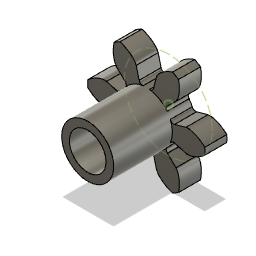
shelf (joined) v52 (Autodesk Fusion 360 archive; units mm, degrees)
design "gear(small)left"
description: small size, for left
description: Spur Gear; Module: 2.0; Num Teeth: 6; Pressure Angle: 20.0; Backlash: 0.00 mm
Autodesk Fusion 360 part; units mm, degrees
(part 1 of 4)
sketch "草图1" plane through (0, 0, 0) normal (0, 0, 1) x (1, 0, 0) in component "Spur Gear (6 teeth)"
  circle A0 centre (0, 0) radius 3.5492
  circle A1 centre (0, 0) radius 2.5
extrude "拉伸1" add sketch "草图1" along normal blind 11 in component "Spur Gear (6 teeth)"
sketch "草图2" plane through (0, 0, 0) normal (0, 0, 1) x (1, 0, 0) in component "Spur Gear (6 teeth)"
  spline S0 degree 5 poles (5.4237, -1.5403) (5.4306, -1.5422) (5.4444, -1.5458) (5.4654, -1.5503) (5.4937, -1.5547) (5.5295, -1.5577) (5.5656, -1.5592) (5.602, -1.5596) (5.6385, -1.5595) (5.6751, -1.559) (5.7117, -1.558) (5.7485, -1.5565) (5.7854, -1.5541) (5.8224, -1.5509) (5.8596, -1.5469) (5.8968, -1.542) (5.9342, -1.5365) (5.9716, -1.5304) (6.009, -1.5238) (6.0465, -1.5167) (6.084, -1.509) (6.1216, -1.5009) (6.1592, -1.4921) (6.1968, -1.4828) (6.2344, -1.473) (6.2721, -1.4625) (6.3098, -1.4516) (6.3475, -1.4402) (6.3851, -1.4282) (6.4228, -1.4158) (6.4605, -1.403) (6.4982, -1.3896) (6.5358, -1.3757) (6.5734, -1.3614) (6.611, -1.3466) (6.6486, -1.3313) (6.6861, -1.3156) (6.7236, -1.2994) (6.7611, -1.2828) (6.7985, -1.2657) (6.8359, -1.2482) (6.8732, -1.2302) (6.9104, -1.2118) (6.9476, -1.193) (6.9848, -1.1737) (7.0219, -1.154) (7.0589, -1.1339) (7.0958, -1.1133) (7.1326, -1.0923) (7.1694, -1.071) (7.2061, -1.0492) (7.2427, -1.027) (7.2792, -1.0043) (7.3157, -0.9813) (7.352, -0.9579) (7.3882, -0.9341) (7.4244, -0.9098) (7.4604, -0.8852) (7.4963, -0.8602) (7.5321, -0.8348) (7.5678, -0.809) (7.6034, -0.7828) (7.6388, -0.7563) (7.6742, -0.7293) (7.7094, -0.702) (7.7445, -0.6743) (7.7794, -0.6462) (7.8142, -0.6178) (7.8489, -0.589) (7.8834, -0.5598) (7.9178, -0.5303) (7.9452, -0.5063) (7.9657, -0.4882) (7.9794, -0.4761) (7.9862, -0.47) knots 0 0 0 0 0 0 0.01428571 0.02857143 0.04285714 0.05714286 0.07142857 0.08571429 0.1 0.11428571 0.12857143 0.14285714 0.15714286 0.17142857 0.18571429 0.2 0.21428571 0.22857143 0.24285714 0.25714286 0.27142857 0.28571429 0.3 0.31428571 0.32857143 0.34285714 0.35714286 0.37142857 0.38571429 0.4 0.41428571 0.42857143 0.44285714 0.45714286 0.47142857 0.48571429 0.5 0.51428571 0.52857143 0.54285714 0.55714286 0.57142857 0.58571429 0.6 0.61428571 0.62857143 0.64285714 0.65714286 0.67142857 0.68571429 0.7 0.71428571 0.72857143 0.74285714 0.75714286 0.77142857 0.78571429 0.8 0.81428571 0.82857143 0.84285714 0.85714286 0.87142857 0.88571429 0.9 0.91428571 0.92857143 0.94285714 0.95714286 0.97142857 0.98571429 1 1 1 1 1 1
  spline S1 degree 5 poles (5.4237, 1.5403) (5.4306, 1.5422) (5.4444, 1.5458) (5.4654, 1.5503) (5.4937, 1.5547) (5.5295, 1.5577) (5.5656, 1.5592) (5.602, 1.5596) (5.6385, 1.5595) (5.6751, 1.559) (5.7117, 1.558) (5.7485, 1.5565) (5.7854, 1.5541) (5.8224, 1.5509) (5.8596, 1.5469) (5.8968, 1.542) (5.9342, 1.5365) (5.9716, 1.5304) (6.009, 1.5238) (6.0465, 1.5167) (6.084, 1.509) (6.1216, 1.5009) (6.1592, 1.4921) (6.1968, 1.4828) (6.2344, 1.473) (6.2721, 1.4625) (6.3098, 1.4516) (6.3475, 1.4402) (6.3851, 1.4282) (6.4228, 1.4158) (6.4605, 1.403) (6.4982, 1.3896) (6.5358, 1.3757) (6.5734, 1.3614) (6.611, 1.3466) (6.6486, 1.3313) (6.6861, 1.3156) (6.7236, 1.2994) (6.7611, 1.2828) (6.7985, 1.2657) (6.8359, 1.2482) (6.8732, 1.2302) (6.9104, 1.2118) (6.9476, 1.193) (6.9848, 1.1737) (7.0219, 1.154) (7.0589, 1.1339) (7.0958, 1.1133) (7.1326, 1.0923) (7.1694, 1.071) (7.2061, 1.0492) (7.2427, 1.027) (7.2792, 1.0043) (7.3157, 0.9813) (7.352, 0.9579) (7.3882, 0.9341) (7.4244, 0.9098) (7.4604, 0.8852) (7.4963, 0.8602) (7.5321, 0.8348) (7.5678, 0.809) (7.6034, 0.7828) (7.6388, 0.7563) (7.6742, 0.7293) (7.7094, 0.702) (7.7445, 0.6743) (7.7794, 0.6462) (7.8142, 0.6178) (7.8489, 0.589) (7.8834, 0.5598) (7.9178, 0.5303) (7.9452, 0.5063) (7.9657, 0.4882) (7.9794, 0.4761) (7.9862, 0.47) knots 0 0 0 0 0 0 0.01428571 0.02857143 0.04285714 0.05714286 0.07142857 0.08571429 0.1 0.11428571 0.12857143 0.14285714 0.15714286 0.17142857 0.18571429 0.2 0.21428571 0.22857143 0.24285714 0.25714286 0.27142857 0.28571429 0.3 0.31428571 0.32857143 0.34285714 0.35714286 0.37142857 0.38571429 0.4 0.41428571 0.42857143 0.44285714 0.45714286 0.47142857 0.48571429 0.5 0.51428571 0.52857143 0.54285714 0.55714286 0.57142857 0.58571429 0.6 0.61428571 0.62857143 0.64285714 0.65714286 0.67142857 0.68571429 0.7 0.71428571 0.72857143 0.74285714 0.75714286 0.77142857 0.78571429 0.8 0.81428571 0.82857143 0.84285714 0.85714286 0.87142857 0.88571429 0.9 0.91428571 0.92857143 0.94285714 0.95714286 0.97142857 0.98571429 1 1 1 1 1 1
  arc A0 (7.9862, -0.47) -> (7.9862, 0.47) centre (0, 0) ccw
  line L0 (3.4046, -0.9696) -> (5.4237, -1.5403)
  line L1 (3.4046, 0.9696) -> (5.4237, 1.5403)
  line L2 (3.4046, -0.9696) -> (3.4046, 0.9696)
  point P0 (5.5935, -1.5594)
  point P1 (5.7697, -1.555)
  point P2 (5.9497, -1.5339)
  point P3 (6.1326, -1.4982)
  point P4 (6.3176, -1.4491)
  point P5 (6.5041, -1.3873)
  point P6 (6.6914, -1.3132)
  point P7 (6.8792, -1.2272)
  point P8 (7.0668, -1.1294)
  point P9 (7.2538, -1.02)
  point P10 (7.4397, -0.8993)
  point P11 (7.6241, -0.7673)
  point P12 (7.8064, -0.6241)
  point P13 (5.5935, 1.5594)
  point P14 (5.7697, 1.555)
  point P15 (5.9497, 1.5339)
  point P16 (6.1326, 1.4982)
  point P17 (6.3176, 1.4491)
  point P18 (6.5041, 1.3873)
  point P19 (6.6914, 1.3132)
  point P20 (6.8792, 1.2272)
  point P21 (7.0668, 1.1294)
  point P22 (7.2538, 1.02)
  point P23 (7.4397, 0.8993)
  point P24 (7.6241, 0.7673)
  point P25 (7.8064, 0.6241)
extrude "拉伸2" add sketch "草图2" along normal blind 3 in component "Spur Gear (6 teeth)"
fillet "圆角1" radius 0.5 2 edges at (3.4135, -0.9721, 1.5) (3.4135, 0.9721, 1.5) in component "Spur Gear (6 teeth)"
pattern_circular "C-阵列1" count 6 over 360 about axis through (0, 0, 0) along (0, 0, 1) of "拉伸2", "圆角1" in component "Spur Gear (6 teeth)"
sketch "草图3" plane through (0, 0, 0) normal (0, 0, 1) x (1, 0, 0) in component "Spur Gear (6 teeth)"
  circle A0 centre (0, 0) radius 6 construction
component "Spur Gear (6 teeth)" placed x (1, 0, 0) y (0, 1, 0) z (0, 0, 1) at (0, 0, 0)

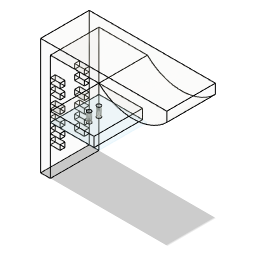
design "clamp"
Autodesk Fusion 360 part; units mm, degrees
sketch "草图1" plane through (0, 0, 0) normal (0, 1, 0) x (1, 0, 0) in component "Component"
  line L0 (-30, 25) -> (30, 25)
  line L1 (30, 25) -> (30, -25)
  line L2 (30, -25) -> (-30, -25)
  line L3 (-30, -25) -> (-30, 25)
  line L4 (-30, 25) -> (30, -25) construction
  line L5 (30, 25) -> (-30, -25) construction
  dimension "d1" = 60
  dimension "d2" = 50
  constraint horizontal L0
  constraint perpendicular L0 L1
  constraint parallel L0 L2
  constraint parallel L1 L3
  constraint coincident L4 origin
  constraint coincident L5 origin
  measures "d1" distance of L0.start L0.end
  measures "d2" distance of L0.start L2.end
extrude "拉伸1" add sketch "草图1" along normal blind 10 makes body 1 in component "Component"
sketch "草图2" plane through (0, 10, 0) normal (0, 1, 0) x (-1, 0, 0) in component "Component"
  line L0 (30, 25) -> (-30, 25)
  line L1 (-30, 25) -> (-30, -25)
  line L2 (-30, -25) -> (30, -25)
  line L3 (30, -25) -> (30, 25)
  line L4 (30, -25) -> (20, -25)
  line L5 (20, -25) -> (20, 25)
  line L6 (20, 25) -> (30, 25)
  line L7 (30, 25) -> (30, -25)
  dimension "d5" = 10
  constraint horizontal L4
  constraint vertical L5
  constraint horizontal L6
  constraint vertical L7
  constraint coincident L0 L5.end
  constraint coincident L2.end L3.start
  measures "d5" distance of L2.end L4.end
extrude "拉伸2" add sketch "草图2" along normal blind 60 contours L0 L2 L3 L4 L5 L6 L7 bodies 1 in component "Component"
sketch "草图3" plane through (-20, 0, 0) normal (1, 0, 0) x (0, 0, -1) in component "Component"
  line L0 (-25, 10) -> (25, 10)
  line L1 (25, 10) -> (25, 70)
  line L2 (25, 70) -> (-25, 70)
  line L3 (-25, 70) -> (-25, 10)
  line L4 (-25, 70) -> (25, 70)
  line L5 (25, 70) -> (25, 60)
  line L6 (25, 60) -> (-25, 60)
  line L7 (-25, 60) -> (-25, 70)
  dimension "d8" = 10
  constraint horizontal L4
  constraint vertical L5
  constraint horizontal L6
  constraint vertical L7
  constraint coincident L1 L5.end
  constraint coincident L2.end L3.start
  measures "d8" distance of L2.end L6.end
extrude "拉伸3" add sketch "草图3" along normal blind 120 contours L1 L2 L3 L4 L5 L6 L7 bodies 1 in component "Component"
sketch "草图1 (2)" plane through (0, 0, 25) normal (0, 0, 1) x (1, 0, 0)
  line L0 (-30, 0) -> (30, 0)
  line L1 (30, 0) -> (30, 10)
  line L2 (30, 10) -> (-20, 10)
  line L3 (-20, 10) -> (-20, 60)
  line L4 (-20, 60) -> (100, 60)
  line L5 (100, 60) -> (100, 70)
  line L6 (100, 70) -> (-30, 70)
  line L7 (-30, 70) -> (-30, 0)
  arc A0 (30, 60) -> (100, 60) centre (65, 95.7071) ccw
  dimension "d14" = 50
  dimension "d15" = 50
  constraint coincident L4.end L5.start
  constraint coincident L4 A0.start
  measures "d14" radius of A0
  measures "d15" distance of L3.end A0.start
extrude "拉伸4" add sketch "草图1 (2)" against normal blind 50 contours L4 A0 bodies 1 in component "Component"
sketch "草图2 (2)" plane through (0, 0, 0) normal (0, -1, 0) x (1, 0, 0)
  line L0 (30, 25) -> (-30, 25)
  line L1 (-30, 25) -> (-30, -25)
  line L2 (-30, -25) -> (30, -25)
  line L3 (30, -25) -> (30, 25)
  line L4 (-20, -25) -> (-20, 25)
  line L5 (-30, 25) -> (-20, 25)
  line L6 (-20, 25) -> (-20, -25)
  line L7 (-20, -25) -> (-30, -25)
  line L8 (-30, -25) -> (-30, 25)
  constraint horizontal L5
  constraint vertical L6
  constraint horizontal L7
  constraint vertical L8
  constraint coincident L4.start L6.end
  constraint coincident L0.end L1.start
extrude "拉伸5" add sketch "草图2 (2)" along normal blind 50 contours L0 L1 L2 L4 L5 L6 L7 L8 bodies 1 in component "Component"
sketch "草图3 (2)" plane through (0, 0, 0) normal (0, -1, 0) x (1, 0, 0)
  line L0 (-20, 25) -> (-20, -25)
  line L1 (-20, -25) -> (30, -25)
  line L2 (30, -25) -> (30, 25)
  line L3 (30, 25) -> (-20, 25)
  dimension "d21" = 20
  measures "d21" distance of origin L0
ref_plane "工作平面2" through (-20, 0, 0) normal (1, 0, 0) x (0, 1, 0)
split "分割1" by plane through (-20, 0, 0) normal (1, 0, 0) bodies 1 makes body 2 at (20, 70, -8.3333) makes body 3 at (-3.3333, 0, -8.3333) in component "Component"
combine "合并1" operation add target body 2 tool bodies 1 in component "Component"
sketch "草图4" plane through (-20, 0, 0) normal (-1, 0, 0) x (0, 0, 1)
  line L0 (25, 10) -> (-25, 10)
  line L1 (-25, 10) -> (-25, 0)
  line L2 (-25, 0) -> (25, 0)
  line L3 (25, 0) -> (25, 10)
  line L4 (-15, 7) -> (-10, 7)
  line L5 (-10, 7) -> (-10, 2)
  line L6 (-10, 2) -> (-15, 2)
  line L7 (-15, 2) -> (-15, 7)
  line L8 (10, 7) -> (15, 7)
  line L9 (15, 7) -> (15, 2)
  line L10 (15, 2) -> (10, 2)
  line L11 (10, 2) -> (10, 7)
  dimension "d24" = 5
  dimension "d25" = 5
  dimension "d26" = 5
  dimension "d27" = 10
  dimension "d28" = 3
  dimension "d29" = 5
  dimension "d30" = 5
  dimension "d31" = 10
  dimension "d32" = 3
  constraint horizontal L4
  constraint vertical L5
  constraint horizontal L6
  constraint vertical L7
  constraint horizontal L8
  constraint vertical L9
  constraint horizontal L10
  constraint vertical L11
  measures "d24" distance of L4.start L4.end
  measures "d25" distance of L4.start L6.end
  measures "d26" distance of L4.start L4.end
  measures "d27" distance of origin L5
  measures "d28" distance of L0 L4
  measures "d29" distance of L8.start L8.end
  measures "d30" distance of L8.start L10.end
  measures "d31" distance of L11 origin
  measures "d32" distance of L0 L8
extrude "拉伸6" add sketch "草图4" along normal blind 8 contours L4 L5 L6 L7 | L8 L9 L10 L11 bodies 3 in component "Component"
sketch "草图5" plane through (-20, 0, 0) normal (1, 0, 0) x (0, 0, -1)
  line L0 (25, 60) -> (-25, 60)
  line L1 (-25, 60) -> (-25, -50)
  line L2 (-25, -50) -> (25, -50)
  line L3 (25, -50) -> (25, 60)
  line L4 (-10, 2) -> (-15, 2)
  line L5 (-15, 2) -> (-15, 7)
  line L6 (-15, 7) -> (-10, 7)
  line L7 (-10, 7) -> (-10, 2)
  line L8 (15, 2) -> (10, 2)
  line L9 (10, 2) -> (10, 7)
  line L10 (10, 7) -> (15, 7)
  line L11 (15, 7) -> (15, 2)
  line L12 (-15, 7) -> (-10, 7)
  line L13 (-10, 7) -> (-10, 2)
  line L14 (-10, 2) -> (-15, 2)
  line L15 (-15, 2) -> (-15, 7)
  line L16 (10, 7) -> (15, 7)
  line L17 (15, 7) -> (15, 2)
  line L18 (15, 2) -> (10, 2)
  line L19 (10, 2) -> (10, 7)
  constraint horizontal L12
  constraint vertical L13
  constraint horizontal L14
  constraint vertical L15
  constraint coincident L4.start L7.end
  constraint coincident L5.end L6.start
  constraint horizontal L16
  constraint vertical L17
  constraint horizontal L18
  constraint vertical L19
  constraint coincident L8.start L11.end
  constraint coincident L9.end L10.start
extrude "拉伸7" cut sketch "草图5" against normal blind 10 contours L4 L5 L6 L7 L12 L13 L14 L15 | L8 L9 L10 L11 L16 L17 L18 L19 bodies 2 in component "Component"
extrude "拉伸8" add 2 faces at (-28, 5.3333, 11.6667) (-28, 5.3333, -13.3333) along direction (-1, 0, 0) blind 2 on bodies 3 bodies 3 in component "Component"
sketch "草图6" plane through (-30, 0, 0) normal (-1, 0, 0) x (0, 0, 1)
  line L0 (10, 2) -> (10, 7)
  line L1 (10, 7) -> (15, 7)
  line L2 (15, 7) -> (15, 2)
  line L3 (15, 2) -> (10, 2)
  line L4 (-15, 2) -> (-15, 7)
  line L5 (-15, 7) -> (-10, 7)
  line L6 (-10, 7) -> (-10, 2)
  line L7 (-10, 2) -> (-15, 2)
  line L8 (25, -50) -> (25, 70)
  line L9 (25, 70) -> (-25, 70)
  line L10 (-25, 70) -> (-25, -50)
  line L11 (-25, -50) -> (25, -50)
  line L12 (-15, 20) -> (-10, 20)
  line L13 (-10, 20) -> (-10, 15)
  line L14 (-10, 15) -> (-15, 15)
  line L15 (-15, 15) -> (-15, 20)
  line L16 (10, 20) -> (15, 20)
  line L17 (15, 20) -> (15, 15)
  line L18 (15, 15) -> (10, 15)
  line L19 (10, 15) -> (10, 20)
  line L20 (-15, 30) -> (-10, 30)
  line L21 (-10, 30) -> (-10, 25)
  line L22 (-10, 25) -> (-15, 25)
  line L23 (-15, 25) -> (-15, 30)
  line L24 (10, 30) -> (15, 30)
  line L25 (15, 30) -> (15, 25)
  line L26 (15, 25) -> (10, 25)
  line L27 (10, 25) -> (10, 30)
  line L28 (-15, -5) -> (-10, -5)
  line L29 (-10, -5) -> (-10, -10)
  line L30 (-10, -10) -> (-15, -10)
  line L31 (-15, -10) -> (-15, -5)
  line L32 (10, -5) -> (15, -5)
  line L33 (15, -5) -> (15, -10)
  line L34 (15, -10) -> (10, -10)
  line L35 (10, -10) -> (10, -5)
  line L36 (-15, -15) -> (-10, -15)
  line L37 (-10, -15) -> (-10, -20)
  line L38 (-10, -20) -> (-15, -20)
  line L39 (-15, -20) -> (-15, -15)
  line L40 (10, -15) -> (15, -15)
  line L41 (15, -15) -> (15, -20)
  line L42 (15, -20) -> (10, -20)
  line L43 (10, -20) -> (10, -15)
  line L44 (-15, -25) -> (-10, -25)
  line L45 (-10, -25) -> (-10, -30)
  line L46 (-10, -30) -> (-15, -30)
  line L47 (-15, -30) -> (-15, -25)
  line L48 (10, -25) -> (15, -25)
  line L49 (15, -25) -> (15, -30)
  line L50 (15, -30) -> (10, -30)
  line L51 (10, -30) -> (10, -25)
  dimension "d39" = 5
  dimension "d40" = 5
  dimension "d41" = 5
  dimension "d42" = 5
  dimension "d43" = 5
  dimension "d44" = 5
  dimension "d45" = 5
  dimension "d46" = 5
  dimension "d47" = 5
  dimension "d48" = 5
  dimension "d49" = 5
  dimension "d50" = 5
  dimension "d51" = 5
  dimension "d52" = 5
  dimension "d53" = 5
  dimension "d54" = 5
  dimension "d55" = 5
  dimension "d56" = 5
  dimension "d57" = 15
  dimension "d58" = 10
  dimension "d59" = 20
  dimension "d60" = 5
  dimension "d61" = 5
  dimension "d62" = 30
  dimension "d64" = 15
  constraint horizontal L12
  constraint vertical L13
  constraint horizontal L14
  constraint vertical L15
  constraint horizontal L16
  constraint vertical L17
  constraint horizontal L18
  constraint vertical L19
  constraint horizontal L20
  constraint vertical L21
  constraint horizontal L22
  constraint vertical L23
  constraint horizontal L24
  constraint vertical L25
  constraint horizontal L26
  constraint vertical L27
  constraint horizontal L28
  constraint vertical L29
  constraint horizontal L30
  constraint vertical L31
  constraint horizontal L32
  constraint vertical L33
  constraint horizontal L34
  constraint vertical L35
  constraint horizontal L36
  constraint vertical L37
  constraint horizontal L38
  constraint vertical L39
  constraint horizontal L40
  constraint vertical L41
  constraint horizontal L42
  constraint vertical L43
  constraint horizontal L44
  constraint vertical L45
  constraint horizontal L46
  constraint vertical L47
  constraint horizontal L48
  constraint vertical L49
  constraint horizontal L50
  constraint vertical L51
  constraint vertical L6.end L21.end
  constraint vertical L6.end L13.end
  constraint vertical L0.end L18.end
  constraint vertical L0.end L26.end
  constraint horizontal L13.end L18.end
  constraint horizontal L21.end L26.end
  constraint vertical L0.start L32.start
  constraint vertical L32.start L40.start
  constraint vertical L42.end L48.start
  constraint vertical L6.end L28.end
  constraint vertical L29.end L36.end
  constraint vertical L37.end L44.end
  constraint horizontal L28.end L32.start
  constraint horizontal L36.end L40.start
  constraint horizontal L44.end L48.start
  measures "d39" distance of L20.start L20.end
  measures "d40" distance of L20.start L22.end
  measures "d41" distance of L24.start L24.end
  measures "d42" distance of L24.end L25.end
  measures "d43" distance of L16.start L16.end
  measures "d44" distance of L16.start L18.end
  measures "d45" distance of L32.start L32.end
  measures "d46" distance of L32.start L34.end
  measures "d47" distance of L28.start L28.end
  measures "d48" distance of L28.start L30.end
  measures "d49" distance of L36.start L36.end
  measures "d50" distance of L36.start L38.end
  measures "d51" distance of L44.start L44.end
  measures "d52" distance of L44.end L45.end
  measures "d53" distance of L48.start L48.end
  measures "d54" distance of L48.start L50.end
  measures "d55" distance of L40.start L40.end
  measures "d56" distance of L40.start L42.end
  measures "d57" distance of origin L14
  measures "d58" distance of L10 L15
  measures "d59" distance of origin L12
  measures "d60" distance of L12 L22
  measures "d61" distance of origin L28
  measures "d62" distance of origin L46
  measures "d64" distance of origin L36
extrude "拉伸9" cut sketch "草图6" against normal blind 10 contours L12 L13 L14 L15 | L16 L17 L18 L19 | L20 L21 L22 L23 | L24 L25 L26 L27 | L28 L29 L30 L31 | L32 L33 L34 L35 | L36 L37 L38 L39 | L40 L41 L42 L43 | L44 L45 L46 L47 | L48 L49 L50 L51 bodies 2 in component "Component"
sketch "草图7" plane through (0, 0, 0) normal (0, -1, 0) x (1, 0, 0)
  circle A0 centre (0, -5) radius 2.5
  circle A1 centre (0, 5) radius 2.5
  line L0 (1.75, 0) -> (22.5, 0)
  dimension "d67" = 5
  dimension "d68" = 5
  dimension "d69" = 10
  constraint symmetric A0 A1 L0
  measures "d67" diameter of A0
  measures "d68" diameter of A1
  measures "d69" distance of A0.centre A1.centre
extrude "拉伸10" cut sketch "草图7" against normal blind 10 bodies 3 in component "Component"
thread "螺纹2" "ISO Metric profile 5.0 M5x0.8 6H" major diameter 5.12 minor diameter 4.234 pitch 0.8 angle 60 resizes the face on face at (2.4969, 6.6667, -5.1246) on bodies 3 in component "Component"
thread "螺纹3" "ISO Metric profile 5.0 M5x0.8 6H" major diameter 5.12 minor diameter 4.234 pitch 0.8 angle 60 resizes the face on face at (2.4969, 6.6667, 4.8754) on bodies 3 in component "Component"
sketch "草图4 (2)" plane through (0, 0, 0) normal (0, -1, 0) x (1, 0, 0) in component "Component"
  line L0 (25, 25) -> (25, -25)
  line L1 (25, 25) -> (30, 25)
  line L2 (30, 25) -> (30, -25)
  line L3 (30, -25) -> (25, -25)
  point P0 (30, -25)
  dimension "d72" = 5
  dimension "d73" = 50
  constraint vertical L0
  constraint perpendicular L0 L1
  constraint coincident P0 L2.end
  constraint perpendicular L1 L2
  constraint perpendicular L0 L3
  measures "d72" distance of L0.end P0
  measures "d73" distance of L0.start L0.end
extrude "拉伸11" cut sketch "草图4 (2)" against normal blind 10 bodies 3 in component "Component"
component "Component" placed x (1, 0, 0) y (0, 1, 0) z (0, 0, 1) at (0, 0, 0)

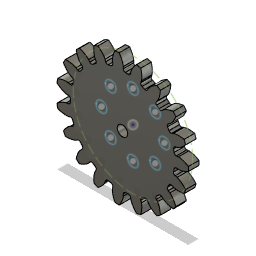
design "gears3"
description: big size
description: Spur Gear; Module: 3.0; Num Teeth: 19; Pressure Angle: 20.0; Backlash: 0.00 mm
Autodesk Fusion 360 part; units mm, degrees
sketch "草图1" plane through (0, 0, 0) normal (0, 0, 1) x (1, 0, 0) in component "Spur Gear (19 teeth)"
  circle A0 centre (0, 0) radius 24.8492
  circle A1 centre (0, 0) radius 2.5
  dimension "d27" = 5
  dimension "d28" = 49.6984
  measures "d27" diameter of A1
  measures "d28" diameter of A0
extrude "拉伸1" add sketch "草图1" along normal blind 5 in component "Spur Gear (19 teeth)"
sketch "草图2" plane through (0, 0, 0) normal (0, 0, 1) x (1, 0, 0) in component "Spur Gear (19 teeth)"
  spline S0 degree 5 poles (26.6538, -2.6091) (26.6677, -2.6105) (26.6955, -2.6128) (26.7371, -2.6152) (26.7928, -2.6162) (26.8625, -2.6145) (26.9323, -2.6108) (27.0021, -2.6057) (27.072, -2.5999) (27.1419, -2.5937) (27.2118, -2.5869) (27.2818, -2.5795) (27.3517, -2.5711) (27.4217, -2.5618) (27.4916, -2.5514) (27.5616, -2.5401) (27.6316, -2.528) (27.7016, -2.5152) (27.7715, -2.5018) (27.8415, -2.4878) (27.9114, -2.4733) (27.9813, -2.4581) (28.0512, -2.4424) (28.121, -2.426) (28.1909, -2.4089) (28.2607, -2.3913) (28.3305, -2.3731) (28.4002, -2.3543) (28.4699, -2.335) (28.5396, -2.3152) (28.6093, -2.2948) (28.6789, -2.274) (28.7485, -2.2526) (28.818, -2.2307) (28.8875, -2.2083) (28.9569, -2.1854) (29.0263, -2.162) (29.0957, -2.1382) (29.165, -2.1138) (29.2342, -2.089) (29.3034, -2.0638) (29.3726, -2.0381) (29.4417, -2.0119) (29.5107, -1.9852) (29.5797, -1.9582) (29.6486, -1.9306) (29.7175, -1.9027) (29.7863, -1.8743) (29.855, -1.8454) (29.9237, -1.8162) (29.9923, -1.7865) (30.0608, -1.7564) (30.1293, -1.7259) (30.1977, -1.695) (30.2661, -1.6637) (30.3343, -1.6319) (30.4025, -1.5998) (30.4707, -1.5672) (30.5387, -1.5343) (30.6067, -1.5009) (30.6746, -1.4672) (30.7424, -1.4331) (30.8102, -1.3986) (30.8778, -1.3637) (30.9454, -1.3284) (31.0129, -1.2928) (31.0803, -1.2567) (31.1477, -1.2203) (31.2149, -1.1836) (31.2821, -1.1464) (31.3492, -1.1089) (31.4028, -1.0786) (31.4429, -1.0557) (31.4697, -1.0404) (31.4831, -1.0327) knots 0 0 0 0 0 0 0.01428571 0.02857143 0.04285714 0.05714286 0.07142857 0.08571429 0.1 0.11428571 0.12857143 0.14285714 0.15714286 0.17142857 0.18571429 0.2 0.21428571 0.22857143 0.24285714 0.25714286 0.27142857 0.28571429 0.3 0.31428571 0.32857143 0.34285714 0.35714286 0.37142857 0.38571429 0.4 0.41428571 0.42857143 0.44285714 0.45714286 0.47142857 0.48571429 0.5 0.51428571 0.52857143 0.54285714 0.55714286 0.57142857 0.58571429 0.6 0.61428571 0.62857143 0.64285714 0.65714286 0.67142857 0.68571429 0.7 0.71428571 0.72857143 0.74285714 0.75714286 0.77142857 0.78571429 0.8 0.81428571 0.82857143 0.84285714 0.85714286 0.87142857 0.88571429 0.9 0.91428571 0.92857143 0.94285714 0.95714286 0.97142857 0.98571429 1 1 1 1 1 1
  spline S1 degree 5 poles (26.6538, 2.6091) (26.6677, 2.6105) (26.6955, 2.6128) (26.7371, 2.6152) (26.7928, 2.6162) (26.8625, 2.6145) (26.9323, 2.6108) (27.0021, 2.6057) (27.072, 2.5999) (27.1419, 2.5937) (27.2118, 2.5869) (27.2818, 2.5795) (27.3517, 2.5711) (27.4217, 2.5618) (27.4916, 2.5514) (27.5616, 2.5401) (27.6316, 2.528) (27.7016, 2.5152) (27.7715, 2.5018) (27.8415, 2.4878) (27.9114, 2.4733) (27.9813, 2.4581) (28.0512, 2.4424) (28.121, 2.426) (28.1909, 2.4089) (28.2607, 2.3913) (28.3305, 2.3731) (28.4002, 2.3543) (28.4699, 2.335) (28.5396, 2.3152) (28.6093, 2.2948) (28.6789, 2.274) (28.7485, 2.2526) (28.818, 2.2307) (28.8875, 2.2083) (28.9569, 2.1854) (29.0263, 2.162) (29.0957, 2.1382) (29.165, 2.1138) (29.2342, 2.089) (29.3034, 2.0638) (29.3726, 2.0381) (29.4417, 2.0119) (29.5107, 1.9852) (29.5797, 1.9582) (29.6486, 1.9306) (29.7175, 1.9027) (29.7863, 1.8743) (29.855, 1.8454) (29.9237, 1.8162) (29.9923, 1.7865) (30.0608, 1.7564) (30.1293, 1.7259) (30.1977, 1.695) (30.2661, 1.6637) (30.3343, 1.6319) (30.4025, 1.5998) (30.4707, 1.5672) (30.5387, 1.5343) (30.6067, 1.5009) (30.6746, 1.4672) (30.7424, 1.4331) (30.8102, 1.3986) (30.8778, 1.3637) (30.9454, 1.3284) (31.0129, 1.2928) (31.0803, 1.2567) (31.1477, 1.2203) (31.2149, 1.1836) (31.2821, 1.1464) (31.3492, 1.1089) (31.4028, 1.0786) (31.4429, 1.0557) (31.4697, 1.0404) (31.4831, 1.0327) knots 0 0 0 0 0 0 0.01428571 0.02857143 0.04285714 0.05714286 0.07142857 0.08571429 0.1 0.11428571 0.12857143 0.14285714 0.15714286 0.17142857 0.18571429 0.2 0.21428571 0.22857143 0.24285714 0.25714286 0.27142857 0.28571429 0.3 0.31428571 0.32857143 0.34285714 0.35714286 0.37142857 0.38571429 0.4 0.41428571 0.42857143 0.44285714 0.45714286 0.47142857 0.48571429 0.5 0.51428571 0.52857143 0.54285714 0.55714286 0.57142857 0.58571429 0.6 0.61428571 0.62857143 0.64285714 0.65714286 0.67142857 0.68571429 0.7 0.71428571 0.72857143 0.74285714 0.75714286 0.77142857 0.78571429 0.8 0.81428571 0.82857143 0.84285714 0.85714286 0.87142857 0.88571429 0.9 0.91428571 0.92857143 0.94285714 0.95714286 0.97142857 0.98571429 1 1 1 1 1 1
  arc A0 (31.4831, -1.0327) -> (31.4831, 1.0327) centre (0, 0) ccw
  line L0 (24.721, -2.4209) -> (26.6538, -2.6091)
  line L1 (24.721, 2.4209) -> (26.6538, 2.6091)
  line L2 (24.721, -2.4209) -> (24.721, 2.4209)
  point P0 (26.9928, -2.6062)
  point P1 (27.3345, -2.573)
  point P2 (27.678, -2.5194)
  point P3 (28.0227, -2.4487)
  point P4 (28.3683, -2.3628)
  point P5 (28.7145, -2.263)
  point P6 (29.0612, -2.15)
  point P7 (29.4081, -2.0245)
  point P8 (29.7549, -1.8871)
  point P9 (30.1016, -1.7382)
  point P10 (30.448, -1.578)
  point P11 (30.7938, -1.4069)
  point P12 (31.1389, -1.225)
  point P13 (26.9928, 2.6062)
  point P14 (27.3345, 2.573)
  point P15 (27.678, 2.5194)
  point P16 (28.0227, 2.4487)
  point P17 (28.3683, 2.3628)
  point P18 (28.7145, 2.263)
  point P19 (29.0612, 2.15)
  point P20 (29.4081, 2.0245)
  point P21 (29.7549, 1.8871)
  point P22 (30.1016, 1.7382)
  point P23 (30.448, 1.578)
  point P24 (30.7938, 1.4069)
  point P25 (31.1389, 1.225)
extrude "拉伸2" add sketch "草图2" along normal blind 5 in component "Spur Gear (19 teeth)"
fillet "圆角1" radius 1 2 edges at (24.7309, -2.4218, 2.5) (24.7309, 2.4218, 2.5) in component "Spur Gear (19 teeth)"
pattern_circular "C-阵列1" count 19 over 360 about axis through (0, 0, 0) along (0, 0, 1) of "拉伸2", "圆角1" in component "Spur Gear (19 teeth)"
sketch "草图3" plane through (0, 0, 0) normal (0, 0, 1) x (1, 0, 0) in component "Spur Gear (19 teeth)"
  circle A0 centre (0, 0) radius 28.5 construction
sketch "Sketch2" plane through (0, 0, 0) normal (0, 1, 0) x (1, 0, 0)
sketch "草图3 (2)" plane through (0, 0, 0) normal (0, 0, -1) x (-1, 0, 0)
  circle A0 centre (0, 0) radius 2.5
  arc A1 (-21.8319, -13.8031) -> (-21.5014, -12.4568) centre (-22.3667, -12.9581) ccw
  line L0 (-21.8319, -13.8031) -> (-22.6362, -14.3122)
  spline S0 degree 5 poles (-22.6362, -14.3122) (-22.648, -14.3196) (-22.6713, -14.3348) (-22.7056, -14.3586) (-22.7502, -14.392) (-22.8041, -14.4361) (-22.8569, -14.4819) (-22.9089, -14.5288) (-22.9605, -14.5763) (-23.0118, -14.6241) (-23.0628, -14.6724) (-23.1135, -14.7212) (-23.1636, -14.7708) (-23.213, -14.8211) (-23.2619, -14.8723) (-23.3102, -14.9242) (-23.3579, -14.9767) (-23.4053, -15.0298) (-23.4522, -15.0834) (-23.4989, -15.1374) (-23.5451, -15.1918) (-23.591, -15.2467) (-23.6365, -15.302) (-23.6815, -15.3579) (-23.7262, -15.4142) (-23.7704, -15.471) (-23.8143, -15.5282) (-23.8578, -15.5859) (-23.901, -15.644) (-23.9438, -15.7024) (-23.9863, -15.7612) (-24.0284, -15.8205) (-24.0702, -15.88) (-24.1116, -15.94) (-24.1527, -16.0004) (-24.1934, -16.0611) (-24.2338, -16.1222) (-24.2739, -16.1836) (-24.3136, -16.2454) (-24.353, -16.3075) (-24.3921, -16.3699) (-24.4309, -16.4327) (-24.4693, -16.4958) (-24.5074, -16.5592) (-24.5452, -16.6229) (-24.5827, -16.687) (-24.6199, -16.7514) (-24.6567, -16.816) (-24.6933, -16.881) (-24.7295, -16.9463) (-24.7654, -17.0118) (-24.801, -17.0777) (-24.8363, -17.1438) (-24.8713, -17.2102) (-24.906, -17.2769) (-24.9404, -17.3439) (-24.9745, -17.4112) (-25.0082, -17.4787) (-25.0417, -17.5465) (-25.0749, -17.6146) (-25.1077, -17.6829) (-25.1403, -17.7515) (-25.1726, -17.8203) (-25.2045, -17.8894) (-25.2362, -17.9588) (-25.2676, -18.0283) (-25.2987, -18.0982) (-25.3294, -18.1683) (-25.3599, -18.2386) (-25.3901, -18.3092) (-25.42, -18.38) (-25.4437, -18.4368) (-25.4613, -18.4796) (-25.473, -18.5081) (-25.4788, -18.5224) knots 0 0 0 0 0 0 0.01428571 0.02857143 0.04285714 0.05714286 0.07142857 0.08571429 0.1 0.11428571 0.12857143 0.14285714 0.15714286 0.17142857 0.18571429 0.2 0.21428571 0.22857143 0.24285714 0.25714286 0.27142857 0.28571429 0.3 0.31428571 0.32857143 0.34285714 0.35714286 0.37142857 0.38571429 0.4 0.41428571 0.42857143 0.44285714 0.45714286 0.47142857 0.48571429 0.5 0.51428571 0.52857143 0.54285714 0.55714286 0.57142857 0.58571429 0.6 0.61428571 0.62857143 0.64285714 0.65714286 0.67142857 0.68571429 0.7 0.71428571 0.72857143 0.74285714 0.75714286 0.77142857 0.78571429 0.8 0.81428571 0.82857143 0.84285714 0.85714286 0.87142857 0.88571429 0.9 0.91428571 0.92857143 0.94285714 0.95714286 0.97142857 0.98571429 1 1 1 1 1 1
  arc A2 (-25.4788, -18.5224) -> (-24.2103, -20.1522) centre (0, 0) ccw
  spline S1 degree 5 poles (-19.4311, -18.4301) (-19.4412, -18.4397) (-19.4617, -18.4586) (-19.4931, -18.486) (-19.5364, -18.521) (-19.5924, -18.5625) (-19.6498, -18.6024) (-19.708, -18.6413) (-19.7667, -18.6797) (-19.8257, -18.7177) (-19.885, -18.7553) (-19.9448, -18.7924) (-20.0051, -18.8288) (-20.0661, -18.8644) (-20.1276, -18.8992) (-20.1898, -18.9332) (-20.2525, -18.9666) (-20.3156, -18.9995) (-20.379, -19.0319) (-20.4428, -19.0638) (-20.5069, -19.0953) (-20.5714, -19.1263) (-20.6362, -19.1568) (-20.7014, -19.1867) (-20.767, -19.2162) (-20.8329, -19.2451) (-20.8992, -19.2736) (-20.9657, -19.3016) (-21.0326, -19.3292) (-21.0998, -19.3564) (-21.1672, -19.3831) (-21.235, -19.4094) (-21.303, -19.4353) (-21.3713, -19.4607) (-21.4399, -19.4857) (-21.5088, -19.5103) (-21.5779, -19.5345) (-21.6473, -19.5583) (-21.7169, -19.5816) (-21.7868, -19.6046) (-21.8569, -19.6271) (-21.9273, -19.6493) (-21.9979, -19.6711) (-22.0687, -19.6925) (-22.1398, -19.7135) (-22.2111, -19.7341) (-22.2826, -19.7543) (-22.3543, -19.7742) (-22.4263, -19.7936) (-22.4985, -19.8127) (-22.5708, -19.8315) (-22.6434, -19.8498) (-22.7162, -19.8678) (-22.7892, -19.8854) (-22.8623, -19.9027) (-22.9357, -19.9195) (-23.0093, -19.9361) (-23.083, -19.9522) (-23.157, -19.968) (-23.2311, -19.9835) (-23.3054, -19.9986) (-23.3799, -20.0133) (-23.4545, -20.0277) (-23.5293, -20.0417) (-23.6043, -20.0554) (-23.6795, -20.0687) (-23.7548, -20.0817) (-23.8303, -20.0943) (-23.906, -20.1066) (-23.9818, -20.1185) (-24.0578, -20.1301) (-24.1187, -20.1391) (-24.1645, -20.1457) (-24.195, -20.1501) (-24.2103, -20.1522) knots 0 0 0 0 0 0 0.01428571 0.02857143 0.04285714 0.05714286 0.07142857 0.08571429 0.1 0.11428571 0.12857143 0.14285714 0.15714286 0.17142857 0.18571429 0.2 0.21428571 0.22857143 0.24285714 0.25714286 0.27142857 0.28571429 0.3 0.31428571 0.32857143 0.34285714 0.35714286 0.37142857 0.38571429 0.4 0.41428571 0.42857143 0.44285714 0.45714286 0.47142857 0.48571429 0.5 0.51428571 0.52857143 0.54285714 0.55714286 0.57142857 0.58571429 0.6 0.61428571 0.62857143 0.64285714 0.65714286 0.67142857 0.68571429 0.7 0.71428571 0.72857143 0.74285714 0.75714286 0.77142857 0.78571429 0.8 0.81428571 0.82857143 0.84285714 0.85714286 0.87142857 0.88571429 0.9 0.91428571 0.92857143 0.94285714 0.95714286 0.97142857 0.98571429 1 1 1 1 1 1
  line L1 (-19.4311, -18.4301) -> (-18.7401, -17.7754)
  arc A3 (-17.3539, -17.7855) -> (-18.7401, -17.7754) centre (-18.0523, -18.5012) ccw
  arc A4 (-17.3539, -17.7855) -> (-16.2917, -18.7634) centre (0, 0) ccw
  arc A5 (-16.1671, -20.144) -> (-16.2917, -18.7634) centre (-16.9473, -19.5184) ccw
  line L2 (-16.1671, -20.144) -> (-16.7625, -20.8867)
  spline S2 degree 5 poles (-16.7625, -20.8867) (-16.7712, -20.8975) (-16.7884, -20.9195) (-16.8132, -20.9531) (-16.8444, -20.9991) (-16.8812, -21.0584) (-16.9162, -21.1188) (-16.9501, -21.1801) (-16.9835, -21.2417) (-17.0165, -21.3037) (-17.0491, -21.3659) (-17.0811, -21.4285) (-17.1124, -21.4916) (-17.1429, -21.5553) (-17.1725, -21.6196) (-17.2013, -21.6843) (-17.2294, -21.7496) (-17.2569, -21.8151) (-17.284, -21.881) (-17.3105, -21.9472) (-17.3366, -22.0137) (-17.3622, -22.0805) (-17.3872, -22.1476) (-17.4117, -22.2151) (-17.4356, -22.2829) (-17.459, -22.351) (-17.482, -22.4194) (-17.5044, -22.488) (-17.5264, -22.557) (-17.5479, -22.6261) (-17.5689, -22.6956) (-17.5896, -22.7653) (-17.6097, -22.8352) (-17.6294, -22.9054) (-17.6487, -22.9758) (-17.6675, -23.0464) (-17.6859, -23.1173) (-17.7038, -23.1884) (-17.7214, -23.2598) (-17.7385, -23.3313) (-17.7552, -23.4031) (-17.7715, -23.475) (-17.7873, -23.5472) (-17.8028, -23.6195) (-17.8179, -23.6921) (-17.8325, -23.7649) (-17.8468, -23.8378) (-17.8606, -23.9109) (-17.8741, -23.9842) (-17.8872, -24.0577) (-17.8998, -24.1314) (-17.9121, -24.2052) (-17.924, -24.2793) (-17.9356, -24.3534) (-17.9467, -24.4278) (-17.9575, -24.5023) (-17.9679, -24.577) (-17.9779, -24.6518) (-17.9875, -24.7268) (-17.9968, -24.8019) (-18.0057, -24.8772) (-18.0142, -24.9527) (-18.0224, -25.0283) (-18.0302, -25.104) (-18.0376, -25.1799) (-18.0447, -25.2559) (-18.0514, -25.332) (-18.0578, -25.4083) (-18.0638, -25.4847) (-18.0694, -25.5613) (-18.0747, -25.638) (-18.0786, -25.6994) (-18.0814, -25.7456) (-18.0832, -25.7764) (-18.0841, -25.7918) knots 0 0 0 0 0 0 0.01428571 0.02857143 0.04285714 0.05714286 0.07142857 0.08571429 0.1 0.11428571 0.12857143 0.14285714 0.15714286 0.17142857 0.18571429 0.2 0.21428571 0.22857143 0.24285714 0.25714286 0.27142857 0.28571429 0.3 0.31428571 0.32857143 0.34285714 0.35714286 0.37142857 0.38571429 0.4 0.41428571 0.42857143 0.44285714 0.45714286 0.47142857 0.48571429 0.5 0.51428571 0.52857143 0.54285714 0.55714286 0.57142857 0.58571429 0.6 0.61428571 0.62857143 0.64285714 0.65714286 0.67142857 0.68571429 0.7 0.71428571 0.72857143 0.74285714 0.75714286 0.77142857 0.78571429 0.8 0.81428571 0.82857143 0.84285714 0.85714286 0.87142857 0.88571429 0.9 0.91428571 0.92857143 0.94285714 0.95714286 0.97142857 0.98571429 1 1 1 1 1 1
  arc A6 (-18.0841, -25.7918) -> (-16.3551, -26.9214) centre (0, 0) ccw
  spline S3 degree 5 poles (-12.394, -23.7408) (-12.4005, -23.7531) (-12.4137, -23.7776) (-12.4345, -23.8138) (-12.4641, -23.8609) (-12.5036, -23.9184) (-12.5449, -23.9747) (-12.5874, -24.0304) (-12.6304, -24.0858) (-12.6739, -24.1409) (-12.7178, -24.1957) (-12.7623, -24.2502) (-12.8075, -24.3042) (-12.8536, -24.3577) (-12.9005, -24.4106) (-12.9483, -24.463) (-12.9967, -24.5149) (-13.0457, -24.5665) (-13.0952, -24.6177) (-13.1451, -24.6686) (-13.1955, -24.7192) (-13.2465, -24.7695) (-13.2979, -24.8194) (-13.3498, -24.8689) (-13.4023, -24.918) (-13.4552, -24.9668) (-13.5086, -25.0153) (-13.5625, -25.0634) (-13.6168, -25.1112) (-13.6715, -25.1587) (-13.7266, -25.2059) (-13.7822, -25.2528) (-13.8381, -25.2993) (-13.8945, -25.3455) (-13.9512, -25.3915) (-14.0084, -25.4371) (-14.0659, -25.4824) (-14.1238, -25.5274) (-14.1821, -25.5721) (-14.2407, -25.6165) (-14.2997, -25.6606) (-14.3591, -25.7044) (-14.4188, -25.748) (-14.4788, -25.7912) (-14.5392, -25.8341) (-14.6, -25.8768) (-14.6611, -25.9191) (-14.7225, -25.9612) (-14.7842, -26.003) (-14.8462, -26.0445) (-14.9086, -26.0857) (-14.9713, -26.1266) (-15.0343, -26.1672) (-15.0976, -26.2076) (-15.1612, -26.2477) (-15.2251, -26.2875) (-15.2893, -26.327) (-15.3538, -26.3662) (-15.4186, -26.4052) (-15.4837, -26.4438) (-15.5491, -26.4822) (-15.6148, -26.5203) (-15.6807, -26.5582) (-15.7469, -26.5957) (-15.8134, -26.633) (-15.8802, -26.6701) (-15.9472, -26.7068) (-16.0145, -26.7433) (-16.0821, -26.7794) (-16.1499, -26.8154) (-16.218, -26.851) (-16.2727, -26.8793) (-16.3139, -26.9004) (-16.3413, -26.9144) (-16.3551, -26.9214) knots 0 0 0 0 0 0 0.01428571 0.02857143 0.04285714 0.05714286 0.07142857 0.08571429 0.1 0.11428571 0.12857143 0.14285714 0.15714286 0.17142857 0.18571429 0.2 0.21428571 0.22857143 0.24285714 0.25714286 0.27142857 0.28571429 0.3 0.31428571 0.32857143 0.34285714 0.35714286 0.37142857 0.38571429 0.4 0.41428571 0.42857143 0.44285714 0.45714286 0.47142857 0.48571429 0.5 0.51428571 0.52857143 0.54285714 0.55714286 0.57142857 0.58571429 0.6 0.61428571 0.62857143 0.64285714 0.65714286 0.67142857 0.68571429 0.7 0.71428571 0.72857143 0.74285714 0.75714286 0.77142857 0.78571429 0.8 0.81428571 0.82857143 0.84285714 0.85714286 0.87142857 0.88571429 0.9 0.91428571 0.92857143 0.94285714 0.95714286 0.97142857 0.98571429 1 1 1 1 1 1
  line L3 (-12.394, -23.7408) -> (-11.9531, -22.8971)
  arc A7 (-10.6387, -22.4566) -> (-11.9531, -22.8971) centre (-11.0668, -23.3604) ccw
  arc A8 (-10.6387, -22.4566) -> (-9.3165, -23.0366) centre (0, 0) ccw
  arc A9 (-8.7504, -24.302) -> (-9.3165, -23.0366) centre (-9.6914, -23.9637) ccw
  line L4 (-8.7504, -24.302) -> (-9.0724, -25.1977)
  spline S4 degree 5 poles (-9.0724, -25.1977) (-9.0771, -25.2109) (-9.0862, -25.2372) (-9.0987, -25.277) (-9.1134, -25.3307) (-9.1289, -25.3987) (-9.1423, -25.4672) (-9.1546, -25.5362) (-9.1661, -25.6053) (-9.1772, -25.6746) (-9.1878, -25.7441) (-9.1978, -25.8137) (-9.2069, -25.8836) (-9.215, -25.9537) (-9.2222, -26.0241) (-9.2284, -26.0947) (-9.2338, -26.1655) (-9.2385, -26.2365) (-9.2427, -26.3076) (-9.2463, -26.3788) (-9.2494, -26.4502) (-9.2519, -26.5216) (-9.2538, -26.5932) (-9.255, -26.665) (-9.2557, -26.7369) (-9.2557, -26.8089) (-9.2552, -26.881) (-9.2541, -26.9532) (-9.2525, -27.0256) (-9.2504, -27.098) (-9.2478, -27.1705) (-9.2446, -27.2431) (-9.241, -27.3158) (-9.2369, -27.3886) (-9.2322, -27.4614) (-9.2271, -27.5344) (-9.2214, -27.6074) (-9.2153, -27.6805) (-9.2087, -27.7536) (-9.2017, -27.8268) (-9.1942, -27.9001) (-9.1862, -27.9735) (-9.1778, -28.0469) (-9.1689, -28.1203) (-9.1596, -28.1938) (-9.1499, -28.2674) (-9.1397, -28.341) (-9.129, -28.4147) (-9.1179, -28.4884) (-9.1064, -28.5622) (-9.0945, -28.636) (-9.0822, -28.7098) (-9.0694, -28.7837) (-9.0562, -28.8576) (-9.0426, -28.9315) (-9.0286, -29.0055) (-9.0142, -29.0795) (-8.9994, -29.1535) (-8.9841, -29.2276) (-8.9685, -29.3017) (-8.9525, -29.3758) (-8.9361, -29.4499) (-8.9192, -29.524) (-8.902, -29.5982) (-8.8844, -29.6724) (-8.8664, -29.7466) (-8.8481, -29.8208) (-8.8293, -29.895) (-8.8102, -29.9692) (-8.7906, -30.0434) (-8.7707, -30.1177) (-8.7545, -30.1771) (-8.7422, -30.2216) (-8.7339, -30.2513) (-8.7297, -30.2662) knots 0 0 0 0 0 0 0.01428571 0.02857143 0.04285714 0.05714286 0.07142857 0.08571429 0.1 0.11428571 0.12857143 0.14285714 0.15714286 0.17142857 0.18571429 0.2 0.21428571 0.22857143 0.24285714 0.25714286 0.27142857 0.28571429 0.3 0.31428571 0.32857143 0.34285714 0.35714286 0.37142857 0.38571429 0.4 0.41428571 0.42857143 0.44285714 0.45714286 0.47142857 0.48571429 0.5 0.51428571 0.52857143 0.54285714 0.55714286 0.57142857 0.58571429 0.6 0.61428571 0.62857143 0.64285714 0.65714286 0.67142857 0.68571429 0.7 0.71428571 0.72857143 0.74285714 0.75714286 0.77142857 0.78571429 0.8 0.81428571 0.82857143 0.84285714 0.85714286 0.87142857 0.88571429 0.9 0.91428571 0.92857143 0.94285714 0.95714286 0.97142857 0.98571429 1 1 1 1 1 1
  arc A10 (-8.7297, -30.2662) -> (-6.7276, -30.7732) centre (0, 0) ccw
  spline S5 degree 5 poles (-4.0139, -26.4787) (-4.016, -26.4925) (-4.0205, -26.52) (-4.0285, -26.561) (-4.0411, -26.6152) (-4.0598, -26.6823) (-4.0806, -26.749) (-4.1027, -26.8155) (-4.1254, -26.8818) (-4.1486, -26.9481) (-4.1724, -27.0142) (-4.1967, -27.0802) (-4.222, -27.1459) (-4.2482, -27.2115) (-4.2754, -27.2767) (-4.3036, -27.3418) (-4.3325, -27.4067) (-4.3621, -27.4713) (-4.3923, -27.5359) (-4.423, -27.6002) (-4.4543, -27.6644) (-4.4861, -27.7285) (-4.5185, -27.7924) (-4.5516, -27.8561) (-4.5852, -27.9196) (-4.6195, -27.9829) (-4.6543, -28.0461) (-4.6896, -28.1091) (-4.7254, -28.172) (-4.7617, -28.2347) (-4.7986, -28.2972) (-4.8359, -28.3596) (-4.8737, -28.4217) (-4.9119, -28.4838) (-4.9507, -28.5456) (-4.9899, -28.6073) (-5.0297, -28.6689) (-5.0698, -28.7302) (-5.1104, -28.7915) (-5.1515, -28.8525) (-5.1929, -28.9134) (-5.2348, -28.9741) (-5.2772, -29.0346) (-5.32, -29.095) (-5.3631, -29.1552) (-5.4067, -29.2153) (-5.4508, -29.2752) (-5.4952, -29.3349) (-5.54, -29.3945) (-5.5852, -29.4539) (-5.6308, -29.5131) (-5.6768, -29.5722) (-5.7232, -29.631) (-5.77, -29.6898) (-5.8171, -29.7483) (-5.8647, -29.8067) (-5.9126, -29.8649) (-5.9608, -29.923) (-6.0095, -29.9809) (-6.0585, -30.0386) (-6.1078, -30.0961) (-6.1576, -30.1535) (-6.2077, -30.2107) (-6.2581, -30.2677) (-6.3089, -30.3246) (-6.36, -30.3813) (-6.4115, -30.4378) (-6.4633, -30.4941) (-6.5155, -30.5503) (-6.568, -30.6063) (-6.6208, -30.6621) (-6.6633, -30.7066) (-6.6954, -30.74) (-6.7168, -30.7621) (-6.7276, -30.7732) knots 0 0 0 0 0 0 0.01428571 0.02857143 0.04285714 0.05714286 0.07142857 0.08571429 0.1 0.11428571 0.12857143 0.14285714 0.15714286 0.17142857 0.18571429 0.2 0.21428571 0.22857143 0.24285714 0.25714286 0.27142857 0.28571429 0.3 0.31428571 0.32857143 0.34285714 0.35714286 0.37142857 0.38571429 0.4 0.41428571 0.42857143 0.44285714 0.45714286 0.47142857 0.48571429 0.5 0.51428571 0.52857143 0.54285714 0.55714286 0.57142857 0.58571429 0.6 0.61428571 0.62857143 0.64285714 0.65714286 0.67142857 0.68571429 0.7 0.71428571 0.72857143 0.74285714 0.75714286 0.77142857 0.78571429 0.8 0.81428571 0.82857143 0.84285714 0.85714286 0.87142857 0.88571429 0.9 0.91428571 0.92857143 0.94285714 0.95714286 0.97142857 0.98571429 1 1 1 1 1 1
  line L5 (-4.0139, -26.4787) -> (-3.8707, -25.5377)
  arc A11 (-2.7706, -24.6943) -> (-3.8707, -25.5377) centre (-2.8821, -25.688) ccw
  arc A12 (-2.7706, -24.6943) -> (-1.3317, -24.8135) centre (0, 0) ccw
  arc A13 (-0.3854, -25.8265) -> (-1.3317, -24.8135) centre (-1.3853, -25.8121) ccw
  line L6 (-0.3854, -25.8265) -> (-0.3991, -26.7783)
  spline S6 degree 5 poles (-0.3991, -26.7783) (-0.3993, -26.7922) (-0.3994, -26.8201) (-0.3983, -26.8618) (-0.3947, -26.9173) (-0.3873, -26.9866) (-0.3778, -27.0559) (-0.367, -27.125) (-0.3554, -27.1942) (-0.3434, -27.2634) (-0.3309, -27.3325) (-0.3177, -27.4016) (-0.3037, -27.4706) (-0.2886, -27.5396) (-0.2725, -27.6084) (-0.2554, -27.6772) (-0.2376, -27.746) (-0.219, -27.8146) (-0.1999, -27.8833) (-0.1802, -27.9518) (-0.1599, -28.0203) (-0.1391, -28.0887) (-0.1176, -28.1571) (-0.0955, -28.2253) (-0.0727, -28.2935) (-0.0494, -28.3616) (-0.0255, -28.4297) (-0.001, -28.4976) (0.024, -28.5655) (0.0495, -28.6333) (0.0755, -28.7011) (0.1021, -28.7687) (0.1291, -28.8363) (0.1567, -28.9038) (0.1847, -28.9712) (0.2133, -29.0385) (0.2423, -29.1057) (0.2718, -29.1729) (0.3018, -29.2399) (0.3322, -29.3069) (0.3631, -29.3738) (0.3945, -29.4405) (0.4263, -29.5072) (0.4585, -29.5738) (0.4912, -29.6403) (0.5243, -29.7068) (0.5579, -29.7731) (0.5919, -29.8393) (0.6263, -29.9054) (0.6611, -29.9714) (0.6963, -30.0374) (0.732, -30.1032) (0.768, -30.1689) (0.8045, -30.2345) (0.8414, -30.3001) (0.8786, -30.3655) (0.9163, -30.4308) (0.9544, -30.496) (0.9928, -30.5611) (1.0317, -30.6261) (1.0709, -30.691) (1.1105, -30.7558) (1.1505, -30.8204) (1.1908, -30.885) (1.2316, -30.9494) (1.2727, -31.0137) (1.3141, -31.078) (1.356, -31.1421) (1.3982, -31.2061) (1.4408, -31.2699) (1.4837, -31.3337) (1.5183, -31.3846) (1.5445, -31.4227) (1.5619, -31.4481) (1.5707, -31.4608) knots 0 0 0 0 0 0 0.01428571 0.02857143 0.04285714 0.05714286 0.07142857 0.08571429 0.1 0.11428571 0.12857143 0.14285714 0.15714286 0.17142857 0.18571429 0.2 0.21428571 0.22857143 0.24285714 0.25714286 0.27142857 0.28571429 0.3 0.31428571 0.32857143 0.34285714 0.35714286 0.37142857 0.38571429 0.4 0.41428571 0.42857143 0.44285714 0.45714286 0.47142857 0.48571429 0.5 0.51428571 0.52857143 0.54285714 0.55714286 0.57142857 0.58571429 0.6 0.61428571 0.62857143 0.64285714 0.65714286 0.67142857 0.68571429 0.7 0.71428571 0.72857143 0.74285714 0.75714286 0.77142857 0.78571429 0.8 0.81428571 0.82857143 0.84285714 0.85714286 0.87142857 0.88571429 0.9 0.91428571 0.92857143 0.94285714 0.95714286 0.97142857 0.98571429 1 1 1 1 1 1
  arc A14 (1.5707, -31.4608) -> (3.629, -31.2903) centre (0, 0) ccw
  spline S7 degree 5 poles (4.8013, -26.3473) (4.8037, -26.3611) (4.8084, -26.3885) (4.8142, -26.4299) (4.8198, -26.4852) (4.8239, -26.5548) (4.8259, -26.6247) (4.8266, -26.6947) (4.8266, -26.7648) (4.8262, -26.835) (4.8252, -26.9052) (4.8236, -26.9756) (4.8211, -27.046) (4.8175, -27.1165) (4.813, -27.1871) (4.8075, -27.2577) (4.8012, -27.3285) (4.7942, -27.3992) (4.7866, -27.4701) (4.7784, -27.5409) (4.7697, -27.6118) (4.7604, -27.6827) (4.7505, -27.7537) (4.7399, -27.8247) (4.7287, -27.8957) (4.7169, -27.9667) (4.7045, -28.0377) (4.6915, -28.1088) (4.678, -28.1799) (4.664, -28.251) (4.6495, -28.3221) (4.6345, -28.3932) (4.6189, -28.4643) (4.6029, -28.5354) (4.5863, -28.6065) (4.5692, -28.6775) (4.5516, -28.7486) (4.5336, -28.8197) (4.5151, -28.8908) (4.4961, -28.9619) (4.4766, -29.0329) (4.4567, -29.1039) (4.4363, -29.175) (4.4154, -29.246) (4.3941, -29.3169) (4.3724, -29.3879) (4.3502, -29.4588) (4.3276, -29.5297) (4.3046, -29.6006) (4.2811, -29.6715) (4.2572, -29.7423) (4.2328, -29.8131) (4.2081, -29.8839) (4.1829, -29.9546) (4.1573, -30.0253) (4.1313, -30.096) (4.1049, -30.1666) (4.0781, -30.2372) (4.0509, -30.3077) (4.0233, -30.3782) (3.9953, -30.4487) (3.9669, -30.5191) (3.9381, -30.5894) (3.9089, -30.6597) (3.8793, -30.73) (3.8494, -30.8002) (3.819, -30.8704) (3.7883, -30.9405) (3.7572, -31.0106) (3.7258, -31.0806) (3.6939, -31.1505) (3.6681, -31.2065) (3.6486, -31.2484) (3.6355, -31.2763) (3.629, -31.2903) knots 0 0 0 0 0 0 0.01428571 0.02857143 0.04285714 0.05714286 0.07142857 0.08571429 0.1 0.11428571 0.12857143 0.14285714 0.15714286 0.17142857 0.18571429 0.2 0.21428571 0.22857143 0.24285714 0.25714286 0.27142857 0.28571429 0.3 0.31428571 0.32857143 0.34285714 0.35714286 0.37142857 0.38571429 0.4 0.41428571 0.42857143 0.44285714 0.45714286 0.47142857 0.48571429 0.5 0.51428571 0.52857143 0.54285714 0.55714286 0.57142857 0.58571429 0.6 0.61428571 0.62857143 0.64285714 0.65714286 0.67142857 0.68571429 0.7 0.71428571 0.72857143 0.74285714 0.75714286 0.77142857 0.78571429 0.8 0.81428571 0.82857143 0.84285714 0.85714286 0.87142857 0.88571429 0.9 0.91428571 0.92857143 0.94285714 0.95714286 0.97142857 0.98571429 1 1 1 1 1 1
  line L7 (4.8013, -26.3473) -> (4.6311, -25.4108)
  arc A15 (5.3977, -24.2559) -> (4.6311, -25.4108) centre (5.615, -25.232) ccw
  arc A16 (5.3977, -24.2559) -> (6.7973, -23.9014) centre (0, 0) ccw
  arc A17 (8.0213, -24.5523) -> (6.7973, -23.9014) centre (7.0709, -24.8633) ccw
  line L8 (8.0213, -24.5523) -> (8.3174, -25.4569)
  spline S8 degree 5 poles (8.3174, -25.4569) (8.3217, -25.4702) (8.3307, -25.4965) (8.3453, -25.5357) (8.3667, -25.587) (8.3962, -25.6502) (8.4277, -25.7126) (8.4604, -25.7745) (8.4938, -25.8362) (8.5276, -25.8977) (8.5619, -25.959) (8.5968, -26.0201) (8.6325, -26.0808) (8.6691, -26.1411) (8.7067, -26.201) (8.7452, -26.2606) (8.7844, -26.3198) (8.8243, -26.3787) (8.8646, -26.4374) (8.9055, -26.4958) (8.9469, -26.554) (8.9889, -26.6119) (9.0314, -26.6696) (9.0745, -26.727) (9.1181, -26.7841) (9.1623, -26.841) (9.207, -26.8975) (9.2522, -26.9539) (9.2979, -27.01) (9.3441, -27.0658) (9.3907, -27.1214) (9.4377, -27.1768) (9.4853, -27.2319) (9.5332, -27.2868) (9.5816, -27.3415) (9.6305, -27.3959) (9.6798, -27.45) (9.7295, -27.5039) (9.7796, -27.5576) (9.8302, -27.6111) (9.8811, -27.6643) (9.9324, -27.7173) (9.9842, -27.77) (10.0363, -27.8226) (10.0888, -27.8749) (10.1417, -27.9269) (10.1949, -27.9788) (10.2486, -28.0303) (10.3026, -28.0817) (10.357, -28.1329) (10.4117, -28.1838) (10.4668, -28.2345) (10.5223, -28.2849) (10.5781, -28.3351) (10.6342, -28.3851) (10.6907, -28.4349) (10.7475, -28.4844) (10.8047, -28.5338) (10.8622, -28.5828) (10.92, -28.6317) (10.9782, -28.6803) (11.0367, -28.7287) (11.0955, -28.7769) (11.1546, -28.8249) (11.2141, -28.8726) (11.2739, -28.9201) (11.3339, -28.9674) (11.3943, -29.0144) (11.455, -29.0612) (11.516, -29.1078) (11.5773, -29.1542) (11.6266, -29.1911) (11.6637, -29.2187) (11.6885, -29.237) (11.7009, -29.2462) knots 0 0 0 0 0 0 0.01428571 0.02857143 0.04285714 0.05714286 0.07142857 0.08571429 0.1 0.11428571 0.12857143 0.14285714 0.15714286 0.17142857 0.18571429 0.2 0.21428571 0.22857143 0.24285714 0.25714286 0.27142857 0.28571429 0.3 0.31428571 0.32857143 0.34285714 0.35714286 0.37142857 0.38571429 0.4 0.41428571 0.42857143 0.44285714 0.45714286 0.47142857 0.48571429 0.5 0.51428571 0.52857143 0.54285714 0.55714286 0.57142857 0.58571429 0.6 0.61428571 0.62857143 0.64285714 0.65714286 0.67142857 0.68571429 0.7 0.71428571 0.72857143 0.74285714 0.75714286 0.77142857 0.78571429 0.8 0.81428571 0.82857143 0.84285714 0.85714286 0.87142857 0.88571429 0.9 0.91428571 0.92857143 0.94285714 0.95714286 0.97142857 0.98571429 1 1 1 1 1 1
  arc A18 (11.7009, -29.2462) -> (13.5923, -28.4165) centre (0, 0) ccw